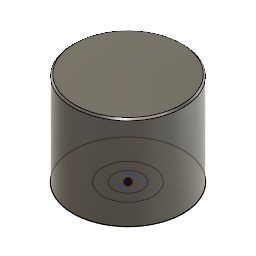
base_stepper_connector v2 (Autodesk Fusion 360 design; units mm, degrees)
Autodesk Fusion 360 part; units mm, degrees
sketch "Sketch1" plane through (0, 0, 0) normal (0, 1, 0) x (1, 0, 0)
  circle A0 centre (0, 0) radius 10
  circle A1 centre (0, 0) radius 4.55
  circle A2 centre (0, 0) radius 2.545
  line L0 (0, 1.52) -> (2.0412, 1.52)
  line L1 (0, 1.52) -> (-2.0412, 1.52)
  line L2 (0, -1.52) -> (-2.0412, -1.52)
  line L3 (0, -1.52) -> (2.0412, -1.52)
  dimension "d1" = 20
  dimension "d2" = 9.1
  dimension "d3" = 5.09
  dimension "d4" = 1.52
  dimension "d6" = 1.52
  measures "d1" diameter of A0
  measures "d2" diameter of A1
  measures "d3" diameter of A2
  measures "d4" distance of A0.centre
  measures "d6" distance of A0.centre
extrude "Extrude1" add sketch "Sketch1" along normal blind 17 contours A0 | A1 | A2 L0 L1 L2 L3 | A2 L0 L1 | A2 L2 L3
extrude "Extrude2" cut sketch "Sketch1" along normal blind 10 contours A2 L0 L1 L2 L3
extrude "Extrude3" cut sketch "Sketch1" along normal blind 4.05 contours A2 L0 L1 | A2 L2 L3
extrude "Extrude4" cut sketch "Sketch1" along normal blind 1.5 contours A1
chamfer "Chamfer1" distance 0.3 angle 45 1 edges at (-9.3233, 17, 3.6162)
